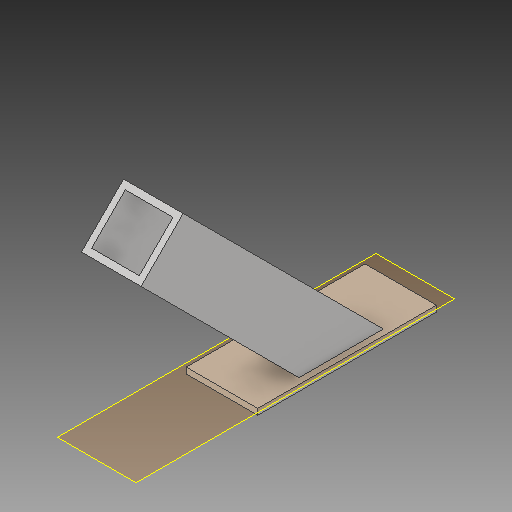
# Autodesk Inventor part: old_design_from_ebay
Saved by Autodesk Inventor 2018 (Build 220112000, 112)
## iProperties
Created: 2018-01-08
Part Number: old_design_from_ebay
Material: Generic
Document SubType Name: Modeling
Designer: erwin
Density: 1 g/cm^3
Appearance: Default
Author: erwin
Autodesk Inventor part; units mm, degrees
ref_plane "YZ Plane" through (0, 0, 0) normal (1, 0, 0) x (0, 1, 0)
ref_plane "XZ Plane" through (0, 0, 0) normal (0, 1, 0) x (-1, 0, 0)
ref_plane "XY Plane" through (0, 0, 0) normal (0, 0, 1) x (1, 0, 0)
sketch "Sketch1" plane through (0, 0, 0) normal (0, 1, 0) x (-1, 0, 0)
  line L0 (12, 30) -> (-12, 30)
  line L1 (-12, 30) -> (-12, -30)
  line L2 (-12, -30) -> (12, -30)
  line L3 (12, -30) -> (12, 30)
  line L4 (12, 30) -> (-12, -30) construction
  line L5 (-12, 30) -> (12, -30) construction
  circle A0 centre (0, 0) radius 4
  dimension "d0" = 24
  dimension "d1" = 60
  dimension "d2" = 8
  constraints: 12 end point, 2 midpoint, 2 parallel, 1 centre point, 1 coincident, 1 horizontal, 1 perpendicular
  measures "d0" distance of L2.end L1.end
  measures "d1" distance of L1.end L0.end
  measures "d2" diameter of A0
extrude "Extrusion1" add sketch "Sketch1" along normal blind 2
sketch "Sketch2" plane through (0, 0, 0) normal (1, 0, 0) x (0, 1, 0)
  line L0 (2, 30) -> (2, -30) projected
  line L1 (2, 0) -> (62.1041, 60.1041)
  line L2 (2, 0) -> (87, 0) construction
  line L3 (69.1751, 53.033) -> (55.033, 67.1751)
  line L4 (69.1751, 53.033) -> (2, -14.1421)
  line L5 (55.033, 67.1751) -> (2, 14.1421)
  line L6 (2, 14.1421) -> (2, -14.1421)
  point P0 (0, 0)
  dimension "d5" = 85
  dimension "d6" = 45
  dimension "d8" = 20
  constraints: 12 end point, 2 point on line, 1 collinear, 1 equal length, 1 horizontal, 1 midpoint, 1 parallel
  measures "d5" distance of L1.start L1.end
  measures "d6" angle of L2 L1
  measures "d8" distance of L3.start L3.end
extrude "Extrusion2" add sketch "Sketch2" along normal mid plane 20
shell "Shell1" thickness 2 removed faces 1 at (1.1806, 2, 0.6196)
move faces "Move1" translate (0, 1.4142, 1.4142) faces at (2.6667, 62.5755, 56.8042)
ref_plane "Work Plane1" through (12, 2, 30) normal (0, 1, 0) x (0, 0, -1)
split body "Split1" result two bodies by plane through (12, 2, 30) normal (0, 1, 0) first body at (3.3333, 46.4299, 30.9948)
equation "\"d9\" = d8"
body "Solid2"
body "Solid3"
